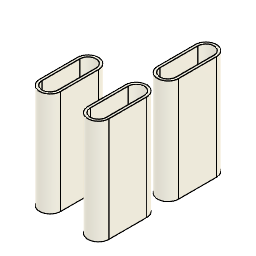
shuffle-cover (Autodesk Fusion 360 design; units mm, degrees)
Autodesk Fusion 360 part; units mm, degrees
sketch "shuffle-cover" plane through (0, 0, 0) normal (0, 0, 1) x (1, 0, 0)
  circle A0 centre (-0.0001, 7.5921) radius 1.1 construction
  line L0 (-3.2401, 2.9921) -> (3.2399, 2.9921) construction
  line L1 (-2.7401, -7.6079) -> (-2.7401, 7.5921)
  arc A1 (3.2399, 7.5921) -> (-3.2401, 7.5921) centre (-0.0001, 7.5921) ccw
  line L2 (3.2399, -7.6079) -> (3.2399, 7.5921)
  arc A2 (-2.7401, -7.6079) -> (2.7399, -7.6079) centre (-0.0001, -7.6079) ccw
  circle A3 centre (-0.0001, -0.0079) radius 1.75 construction
  arc A4 (-3.2401, -7.6079) -> (3.2399, -7.6079) centre (-0.0001, -7.6079) ccw
  circle A5 centre (-0.0001, 7.5921) radius 1.9 construction
  line L3 (2.7399, -7.6079) -> (2.7399, 7.5921)
  line L4 (-3.2401, -7.6079) -> (-3.2401, 7.5921)
  arc A6 (2.7399, 7.5921) -> (-2.7401, 7.5921) centre (-0.0001, 7.5921) ccw
  circle A7 centre (-0.0001, -7.6079) radius 1.9 construction
  circle A8 centre (-0.0001, -7.6079) radius 1.1 construction
  circle A9 centre (-0.0001, -0.0079) radius 1.35 construction
  line L5 (-3.2401, -3.0079) -> (3.2399, -3.0079) construction
  line L6 (-23.64, -7.6) -> (-23.64, 7.6)
  circle A10 centre (-19.4, -7.6) radius 1.9
  arc A11 (-15.16, 7.6) -> (-23.64, 7.6) centre (-19.4, 7.6) ccw
  circle A12 centre (-19.4, 7.6) radius 1.1
  line L7 (-22.64, -3) -> (-16.16, -3)
  arc A13 (-23.64, -7.6) -> (-15.16, -7.6) centre (-19.4, -7.6) ccw
  arc A14 (-16.16, 7.6) -> (-22.64, 7.6) centre (-19.4, 7.6) ccw
  line L8 (-22.64, -7.6) -> (-22.64, 7.6)
  arc A15 (-22.64, -7.6) -> (-16.16, -7.6) centre (-19.4, -7.6) ccw
  circle A16 centre (-19.4, 0) radius 1.35
  circle A17 centre (-19.4, 0) radius 1.75
  line L9 (-16.16, -7.6) -> (-16.16, 7.6)
  circle A18 centre (-19.4, 7.6) radius 1.9
  line L10 (-15.16, -7.6) -> (-15.16, 7.6)
  circle A19 centre (-19.4, -7.6) radius 1.1
  line L11 (-22.64, 3) -> (-16.16, 3)
  arc A20 (3.6399, 7.5921) -> (-3.6401, 7.5921) centre (-0.0001, 7.5921) ccw
  line L12 (-3.6401, -7.6079) -> (-3.6401, 7.5921)
  arc A21 (-3.6401, -7.6079) -> (3.6399, -7.6079) centre (-0.0001, -7.6079) ccw
  line L13 (3.6399, -7.6079) -> (3.6399, 7.5921)
  arc A22 (4.2399, 7.5921) -> (-4.2401, 7.5921) centre (-0.0001, 7.5921) ccw
  line L14 (-4.2401, -7.6079) -> (-4.2401, 7.5921)
  arc A23 (-4.2401, -7.6079) -> (4.2399, -7.6079) centre (-0.0001, -7.6079) ccw
  line L15 (4.2399, -7.6079) -> (4.2399, 7.5921)
  arc A24 (-15.76, 7.6) -> (-23.04, 7.6) centre (-19.4, 7.6) ccw
  line L16 (-23.04, -7.6) -> (-23.04, 7.6)
  arc A25 (-23.04, -7.6) -> (-15.76, -7.6) centre (-19.4, -7.6) ccw
  line L17 (-15.76, -7.6) -> (-15.76, 7.6)
  circle A26 centre (-0.0001, 20.3921) radius 1.1 construction
  circle A27 centre (-0.0001, 20.3921) radius 1.9 construction
  line L18 (3.2399, 20.3921) -> (3.2399, 35.5921)
  line L19 (-3.6401, 20.3921) -> (-3.6401, 35.5921) construction
  arc A28 (3.2399, 35.5921) -> (-3.2401, 35.5921) centre (-0.0001, 35.5921) ccw
  line L20 (-3.2401, 20.3921) -> (-3.2401, 35.5921)
  line L21 (-4.2401, 20.3921) -> (-4.2401, 35.5921)
  arc A29 (2.7399, 35.5921) -> (-2.7401, 35.5921) centre (-0.0001, 35.5921) ccw
  line L22 (-2.7401, 20.3921) -> (-2.7401, 35.5921)
  circle A30 centre (-0.0001, 35.5921) radius 1.9 construction
  line L23 (4.2399, 20.3921) -> (4.2399, 35.5921)
  line L24 (3.6399, 20.3921) -> (3.6399, 35.5921) construction
  circle A31 centre (-0.0001, 35.5921) radius 1.1 construction
  line L25 (2.7399, 20.3921) -> (2.7399, 35.5921)
  arc A32 (4.2399, 35.5921) -> (-4.2401, 35.5921) centre (-0.0001, 35.5921) ccw
  arc A33 (3.6399, 35.5921) -> (-3.6401, 35.5921) centre (-0.0001, 35.5921) ccw construction
  line L26 (-3.2401, 24.9921) -> (3.2399, 24.9921) construction
  arc A34 (-3.2401, 20.3921) -> (3.2399, 20.3921) centre (-0.0001, 20.3921) ccw
  arc A35 (-3.6401, 20.3921) -> (3.6399, 20.3921) centre (-0.0001, 20.3921) ccw construction
  line L27 (-3.2401, 30.9921) -> (3.2399, 30.9921) construction
  arc A36 (-4.2401, 20.3921) -> (4.2399, 20.3921) centre (-0.0001, 20.3921) ccw
  arc A37 (-2.7401, 20.3921) -> (2.7399, 20.3921) centre (-0.0001, 20.3921) ccw
  circle A38 centre (-0.0001, 27.9921) radius 1.75 construction
  circle A39 centre (-0.0001, 27.9921) radius 1.35 construction
  point P0 (-0.0001, -0.0079)
  point P1 (-0.0001, -0.0079)
  point P2 (-19.4, 0)
  point P3 (-19.4, 0)
  point P4 (-0.0001, 27.9921)
  point P5 (-0.0001, 27.9921)
  dimension "d1" = 2.7
  dimension "d2" = 3.8
  dimension "d3" = 2.2
  dimension "d4" = 3.8
  dimension "d5" = 2.2
  dimension "d6" = 3.5
  dimension "d7" = 2.7
  dimension "d8" = 3.8
  dimension "d9" = 2.2
  dimension "d10" = 3.8
  dimension "d11" = 2.2
  dimension "d12" = 3.5
  dimension "d125" = 2.7
  dimension "d126" = 3.8
  dimension "d127" = 2.2
  dimension "d128" = 3.8
  dimension "d129" = 2.2
  dimension "d130" = 3.5
  constraint coincident P1 P0
  constraint concentric A7 A8
  constraint concentric A0 A5
  constraint concentric A3 A9
  constraint coincident L0.end L2
  constraint perpendicular L0 L2
  constraint coincident L5.end L2
  constraint perpendicular L2 L5
  constraint coincident L0.start L4
  constraint coincident L5.start L4
  constraint concentric A1 A6
  constraint concentric A2 A4
  constraint coincident P3 P2
  constraint concentric A10 A19
  constraint concentric A12 A18
  constraint concentric A16 A17
  constraint concentric A11 A14
  constraint concentric A13 A15
  constraint coincident L11.end L9
  constraint perpendicular L9 L11
  constraint coincident L7.end L9
  constraint perpendicular L7 L9
  constraint coincident L11.start L8
  constraint coincident L7.start L8
  constraint concentric A1 A20
  constraint concentric A4 A21
  constraint concentric A1 A22
  constraint concentric A4 A23
  constraint concentric A14 A24
  constraint concentric A15 A25
  constraint coincident P5 P4
  constraint concentric A26 A27
  constraint concentric A30 A31
  constraint concentric A38 A39
  constraint coincident L27.end L18
  constraint perpendicular L18 L27
  constraint coincident L26.end L18
  constraint perpendicular L18 L26
  constraint coincident L27.start L20
  constraint coincident L26.start L20
  constraint concentric A28 A29
  constraint concentric A34 A37
  constraint concentric A28 A33
  constraint concentric A34 A35
  constraint concentric A28 A32
  constraint concentric A34 A36
  measures "d1" diameter of A9
  measures "d2" diameter of A7
  measures "d3" diameter of A8
  measures "d4" diameter of A5
  measures "d5" diameter of A0
  measures "d6" diameter of A3
  measures "d7" diameter of A16
  measures "d8" diameter of A10
  measures "d9" diameter of A19
  measures "d10" diameter of A18
  measures "d11" diameter of A12
  measures "d12" diameter of A17
  measures "d125" diameter of A39
  measures "d126" diameter of A27
  measures "d127" diameter of A26
  measures "d128" diameter of A30
  measures "d129" diameter of A31
  measures "d130" diameter of A38
extrude "Extrude24" add sketch "shuffle-cover" along normal blind 2 contours A10 | L7 L8 A15 L9 | A14 L8 L9 L11 | A18 makes body 1 at (-19.4274, -4.1677, 0) makes body 2 at (-19.3726, 4.1677, 0)
extrude "Extrude25" add sketch "shuffle-cover" along normal blind 1.6 contours L7 L8 L9 L11 | A17 bodies 1 2
extrude "Extrude26" add sketch "shuffle-cover" along normal blind 31.1 contours A24 L16 A25 L17 bodies 1
extrude "Extrude27" add sketch "shuffle-cover" along normal blind 10.1 from surface at 31.7 separate body contours A24 L16 A25 L17 makes body 3
chamfer "Chamfer13" distance 0.4 angle 45 8 edges at (-22.64, 0, 31.7) (-19.4, 10.84, 31.7) (-16.16, 0, 31.7) (-19.4, -10.84, 31.7) (-22.64, 0, 31.1) (-19.4, 10.84, 31.1) (-16.16, 0, 31.1) (-19.4, -10.84, 31.1) measured on face at (-22.64, -1, 35.0667) measured on face at (-20.2775, 10.7189, 35.0667) measured on face at (-16.16, -1, 35.0667) measured on face at (-17.2561, -10.0293, 38.4333) measured on face at (-16.0267, -2.5333, 31.1) measured on face at (-16.0267, -2.5333, 31.1) measured on face at (-16.0267, -2.5333, 31.1) measured on face at (-16.0267, -2.5333, 31.1) on bodies 1 3
extrude "Extrude28" add sketch "shuffle-cover" along normal blind 41.8 contours L6 A11 A13 L10 bodies 1 3
extrude "Extrude29" cut sketch "shuffle-cover" along normal blind 0.3 contours A10 | A17 | A18 bodies 1
chamfer "Chamfer14" distance 0.8 angle 45 2 edges at (-19.7978, -8.6256, 0.3) (-19.7978, 6.5744, 0.3) measured on face at (-18.3055, -7.7095, 0.8667) measured on face at (-19.6979, 8.6589, 0.8667) on bodies 1
chamfer "Chamfer15" distance 0.4 angle 45 1 edges at (-19.8882, -1.2586, 0.3) measured on face at (-18.0567, -0.1344, 0.7333) on bodies 1
extrude "Extrude30" add sketch "shuffle-cover" along normal blind 1 from surface at 1.2 separate body contours A1 L2 A4 L4 makes body 4
chamfer "Chamfer16" distance 0.5 angle 45 4 edges at (2.7399, -0.0079, 1.2) (-0.0001, -10.3479, 1.2) (-2.7401, -0.0079, 1.2) (-0.0001, 10.3321, 1.2) measured on face at (2.7399, 2.5254, 1.8667) measured on face at (2.5746, -8.545, 1.8667) measured on face at (-2.7401, -2.5412, 1.5333) measured on face at (-2.7367, 7.7287, 1.8667) on bodies 4
extrude "Extrude31" add sketch "shuffle-cover" along normal blind 31.3 contours A20 L12 A21 L13 bodies 4
extrude "Extrude32" add sketch "shuffle-cover" along normal blind 10.1 from surface at 31.9 separate body contours A20 L12 A21 L13 makes body 5
chamfer "Chamfer17" distance 0.4 angle 45 8 edges at (-3.2401, -0.0079, 31.9) (-0.0001, 10.8321, 31.9) (3.2399, -0.0079, 31.9) (-0.0001, -10.8479, 31.9) (-3.2401, -0.0079, 31.3) (-0.0001, 10.8321, 31.3) (3.2399, -0.0079, 31.3) (-0.0001, -10.8479, 31.3) measured on face at (-3.2401, -2.5412, 35.2667) measured on face at (-3.224, 7.9147, 38.6333) measured on face at (3.2399, -2.5412, 35.2667) measured on face at (3.2359, -7.7694, 38.6333) measured on face at (-3.3734, 2.5254, 31.3) measured on face at (-3.3734, 2.5254, 31.3) measured on face at (-3.3734, 2.5254, 31.3) measured on face at (-3.3734, 2.5254, 31.3) on bodies 4 5
extrude "Extrude33" add sketch "shuffle-cover" along normal blind 42 contours A22 L14 A23 L15 bodies 4 5
extrude "Extrude34" add sketch "shuffle-cover" along normal blind 1 from surface at 1.2 separate body contours L18 A28 L20 A34 makes body 6
chamfer "Chamfer18" distance 0.5 angle 45 4 edges at (-2.7401, 27.9921, 1.2) (-0.0001, 38.3321, 1.2) (2.7399, 27.9921, 1.2) (-0.0001, 17.6521, 1.2) measured on face at (-2.7401, 25.4588, 1.5333) measured on face at (-2.3381, 37.0208, 1.5333) measured on face at (2.7399, 25.4588, 1.5333) measured on face at (-2.6554, 19.716, 1.8667) on bodies 6
extrude "Extrude35" add sketch "shuffle-cover" along normal blind 42 contours L21 L23 A32 A36 bodies 6
named bodies: "cover-v1-1", "cover-v2-1", "cover-v2-2"
